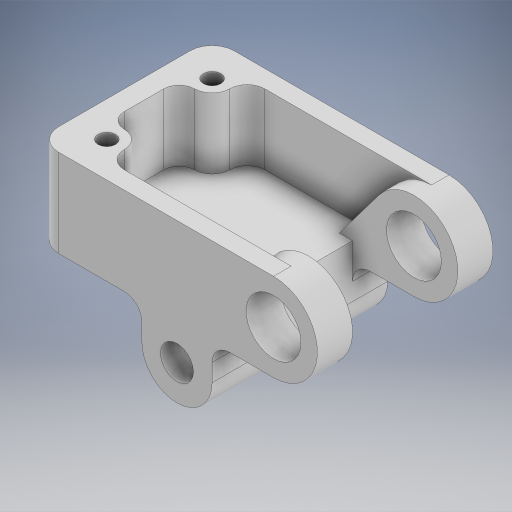
# Autodesk Inventor part: LE-2.2
Saved by Autodesk Inventor 2024 (Build 280153000, 153)
## iProperties
Created: 2024-02-01
Part Number: LE-2.2
Material: Generic
Document SubType Name: Modeling
Designer: Alex
Density: 1 g/cm^3
Appearance: Default
Author: Alex
Autodesk Inventor part; units mm, degrees
ref_plane "YZ Plane" through (0, 0, 0) normal (1, 0, 0) x (0, 1, 0)
ref_plane "XZ Plane" through (0, 0, 0) normal (0, 1, 0) x (-1, 0, 0)
ref_plane "XY Plane" through (0, 0, 0) normal (0, 0, 1) x (1, 0, 0)
sketch "Sketch1" plane through (0, 0, 0) normal (0, 0, 1) x (1, 0, 0)
  line L0 (0, 0) -> (128, 0)
  line L1 (128, 0) -> (128, -40)
  line L2 (128, -40) -> (0, -40)
  line L3 (0, -40) -> (0, 0)
  line L4 (0, -8) -> (-8, -8)
  line L5 (-8, -8) -> (-8, -40)
  line L6 (-8, -40) -> (0, -40)
  line L7 (0, -40) -> (0, -8)
  line L8 (64, 0) -> (64, -40) construction
  line L9 (0, -20) -> (128, -20) construction
  line L10 (48, -40) -> (80, -40)
  line L11 (80, -40) -> (80, -72)
  line L12 (80, -72) -> (48, -72)
  line L13 (48, -72) -> (48, -40)
  line L14 (48, -40) -> (80, -72) construction
  line L15 (80, -40) -> (48, -72) construction
  circle A0 centre (64, -56) radius 7.5
  circle A1 centre (108, -20) radius 12.5
  point P0 (64, -20)
  dimension "d0" = 128
  dimension "d1" = 40
  dimension "d2" = 32
  dimension "d3" = 8
  dimension "d4" = 32
  dimension "d5" = 32
  dimension "d6" = 72
  dimension "d7" = 15
  dimension "d8" = 25
  dimension "d9" = 44
  constraints: 32 end point, 8 midpoint, 6 parallel, 4 point on line, 3 horizontal, 3 perpendicular, 2 centre point, 1 coincident, 1 collinear
  measures "d0" distance of L1.end L2.end
  measures "d1" distance of L0.end L1.end
  measures "d2" distance of L4.end L5.end
  measures "d3" distance of L4.start L4.end
  measures "d4" distance of L11.end L12.end
  measures "d5" distance of L10.end L11.end
  measures "d6" distance between parallel lines of L8 L5
  measures "d7" diameter of A0
  measures "d8" diameter of A1
  measures "d9" distance of A1.centre point (64, -20)
extrude "Extrusion1" add sketch "Sketch1" along normal mid plane 80 contours L0 L1 L2 L3 | L11 L12 L13 L2
extrude "Extrusion2" add sketch "Sketch1" along normal mid plane 32 contours L3 L6 L5 L4
fillet "Fillet1" radius 16 4 edges at (-4, -8, 16) (-4, -8, -16) (48, -72, 0) (80, -72, 0)
fillet "Fillet2" radius 8 2 edges at (80, -40, 0) (48, -40, 0)
fillet "Fillet3" radius 10 2 edges at (0, -20, 40) (0, -20, -40)
sketch "Sketch2" plane through (-8, -40, -16) normal (-1, 0, 0) x (0, 0, 1)
  arc A0 (32, 16) -> (0, 16) centre (16, 16) ccw projected
  line L0 (0, 0) -> (0, 16) projected
  line L1 (0, 0) -> (32, 0) projected
  line L2 (32, 16) -> (32, 0) projected
  circle A1 centre (16, 16) radius 4
  point P0 (16, 40)
  dimension "d17" = 8
  constraints: 1 centre point, 1 coincident
  measures "d17" diameter of A1
extrude "Extrusion3" cut sketch "Sketch2" against normal blind 8 contours A1
sketch "Sketch3" plane through (128, 0, 40) normal (0, 1, 0) x (1, 0, 0)
  arc A0 (-118, 80) -> (-128, 70) centre (-118, 70) ccw projected
  line L0 (-128, 70) -> (-128, 10) projected
  arc A1 (-128, 10) -> (-118, 0) centre (-118, 10) ccw projected
  line L1 (0, 0) -> (-118, 0) projected
  line L2 (0, 0) -> (0, 80) projected
  line L3 (-118, 80) -> (0, 80) projected
  line L4 (-128, 40) -> (0, 40) construction
  circle A2 centre (-112, 16) radius 4
  circle A3 centre (-112, 64) radius 4
  dimension "d20" = 8
  dimension "d21" = 16
  dimension "d22" = 16
  constraints: 2 centre point, 2 end point, 1 midpoint, 1 symmetric about line, 1 other
  measures "d20" diameter of A2
  measures "d21" distance from line of L0 A2.centre
  measures "d22" distance from line of L1 A2.centre
extrude "Extrusion4" cut sketch "Sketch3" against normal through all contours A2 | A3
sketch "Sketch4" plane through (128, 0, 40) normal (0, 1, 0) x (1, 0, 0)
  circle A0 centre (-112, 16) radius 4 construction
  circle A1 centre (-112, 64) radius 4 construction
  arc A2 (-118, 80) -> (-128, 70) centre (-118, 70) ccw construction
  line L0 (-128, 70) -> (-128, 10) construction
  arc A3 (-128, 10) -> (-118, 0) centre (-118, 10) ccw construction
  line L1 (0, 0) -> (-118, 0) construction
  line L2 (0, 0) -> (0, 80) construction
  line L3 (-118, 80) -> (0, 80) construction
  line L4 (-128, 40) -> (0, 40) construction
  line L5 (-112, 16) -> (0, 16) construction
  line L6 (0, 16) -> (0, 64) construction
  line L7 (0, 64) -> (-112, 64) construction
  line L8 (-112, 64) -> (-112, 16) construction
  line L9 (-48, 40) -> (-48, 8)
  line L10 (-48, 8) -> (-96, 8)
  line L11 (-96, 8) -> (-104, 8)
  line L12 (-104, 24) -> (-112, 24)
  line L13 (-119, 40) -> (-119, 24)
  line L14 (-112, 24) -> (-119, 24)
  line L15 (-104, 8) -> (-104, 16)
  line L16 (-104, 16) -> (-104, 24)
  line L17 (-48, 40) -> (-48, 72)
  line L18 (-48, 72) -> (-96, 72)
  line L19 (-96, 72) -> (-104, 72)
  line L20 (-104, 56) -> (-112, 56)
  line L21 (-119, 40) -> (-119, 56)
  line L22 (-112, 56) -> (-119, 56)
  line L23 (-104, 72) -> (-104, 64)
  line L24 (-104, 64) -> (-104, 56)
  dimension "d25" = 8
  dimension "d26" = 48
  dimension "d28" = 8
  dimension "d29" = 8
  dimension "d31" = 16
  dimension "d32" = 9
  dimension "d34" = 8
  constraints: 42 end point, 7 point on line, 7 symmetric about line, 5 perpendicular, 4 horizontal, 2 parallel, 1 midpoint
  measures "d25" distance from line of L1 L9.end
  measures "d26" distance between parallel lines of L2 L9
  measures "d28" distance of L10.end L11.end
  measures "d29" distance of L12.start L12.end
  measures "d31" distance between parallel lines of L3 L7
  measures "d32" distance between parallel lines of L13 L0
  measures "d34" distance of L15.end L12.start
extrude "Extrusion5" cut sketch "Sketch4" against normal blind 32
fillet "Fillet4" radius 8 4 edges at (24, -16, 32) (24, -16, 16) (24, -16, -16) (24, -16, -32)
fillet "Fillet5" radius 7 2 edges at (9, -16, -16) (9, -16, 16)
sketch "Sketch5" plane through (128, 0, 40) normal (0, 1, 0) x (1, 0, 0)
  arc A0 (-112, 56) -> (-104, 64) centre (-112, 64) ccw construction
  arc A1 (-96, 72) -> (-104, 64) centre (-96, 64) ccw construction
  line L0 (-96, 72) -> (-48, 72) construction
  line L1 (-48, 72) -> (-48, 8) construction
  line L2 (-48, 8) -> (-96, 8) construction
  arc A2 (-104, 16) -> (-96, 8) centre (-96, 16) ccw construction
  arc A3 (-104, 16) -> (-112, 24) centre (-112, 16) ccw construction
  arc A4 (-119, 31) -> (-112, 24) centre (-112, 31) ccw construction
  line L3 (-119, 31) -> (-119, 49) construction
  arc A5 (-112, 56) -> (-119, 49) centre (-112, 49) ccw construction
  circle A6 centre (-112, 16) radius 4 construction
  circle A7 centre (-112, 64) radius 4 construction
  arc A8 (-118, 80) -> (-128, 70) centre (-118, 70) ccw construction
  line L4 (-128, 70) -> (-128, 10) construction
  arc A9 (-128, 10) -> (-118, 0) centre (-118, 10) ccw construction
  line L5 (0, 0) -> (-118, 0) construction
  line L6 (0, 0) -> (0, 80) construction
  line L7 (-118, 80) -> (0, 80) construction
  line L8 (-128, 40) -> (0, 40) construction
  line L9 (-48, 16) -> (0, 16)
  line L10 (0, 16) -> (0, 64)
  line L11 (0, 64) -> (-48, 64)
  line L12 (-48, 64) -> (-48, 16)
  line L13 (-48, 16) -> (0, 64) construction
  line L14 (0, 16) -> (-48, 64) construction
  line L15 (-48, 72) -> (-48, 8) projected
  point P0 (-24, 40)
  dimension "d39" = 16
  constraints: 14 end point, 3 midpoint, 3 point on line, 2 parallel, 1 horizontal, 1 perpendicular
  measures "d39" distance between parallel lines of L7 L11
extrude "Extrusion6" cut sketch "Sketch5" against normal through all
fillet "Fillet6" radius 20 4 edges at (128, 0, 32) (128, -40, 32) (128, 0, -32) (128, -40, -32)
sketch "Sketch6" plane through (80, -32, -24) normal (0, 0, 1) x (1, 0, 0)
  arc A0 (28, -8) -> (28, 32) centre (28, 12) ccw construction
  line L0 (28, -8) -> (8, -8) construction
  arc A1 (8, -8) -> (0, -16) centre (8, -16) ccw construction
  line L1 (0, -16) -> (0, -24) construction
  arc A2 (-32, -24) -> (0, -24) centre (-16, -24) ccw construction
  line L2 (-32, -24) -> (-32, -16) construction
  arc A3 (-32, -16) -> (-40, -8) centre (-40, -16) ccw construction
  line L3 (-40, -8) -> (-70, -8) construction
  line L4 (-70, 32) -> (-70, -8) construction
  line L5 (-70, 32) -> (28, 32) construction
  circle A4 centre (-16, -24) radius 7.5 construction
  circle A5 centre (28, 12) radius 12.5 projected
  line L6 (28, 12) -> (28, 32) construction
  line L7 (28, 12) -> (48, 12) construction
  arc A6 (28, 32) -> (12.0273, 24.0363) centre (28, 12) ccw
  line L8 (-48, 0) -> (-48, 32) construction
  line L9 (-48, 0) -> (0, 0) construction
  line L10 (0, 32) -> (0, 0) construction
  line L11 (-48, 32) -> (0, 32) construction
  line L12 (-6.0854, 0) -> (12.0273, 24.0363)
  line L13 (-48, 0) -> (0, 0) projected
  line L14 (-6.0854, 0) -> (0, 0)
  line L15 (0, 0) -> (0, 32)
  line L16 (-70, 32) -> (28, 32) projected
  line L17 (0, 32) -> (28, 32)
  point P0 (-80, 32)
  point P1 (0, 8.0755)
  dimension "d43" = 53
  constraints: 12 end point, 3 point on circle, 2 collinear, 1 centre point, 1 coincident, 1 horizontal, 1 point on line, 1 tangent, 1 vertical
  measures "d43" angle of L9 L12
extrude "Extrusion7" cut sketch "Sketch6" against normal blind 8 contours A6 L12 L15 L16
extrude "Extrusion8" add sketch "Sketch6" against normal blind 8 contours L15 L13 L12
mirror "Mirror1" about plane through (0, 0, 0) normal (0, 0, 1) of "Extrusion7", "Extrusion8"
body "Solid1"
